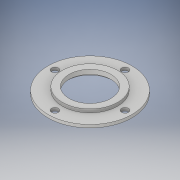
# Autodesk Inventor part: Flange_1
Saved by Autodesk Inventor 2019.4 (Build 234330000, 330)
## iProperties
Created: 2021-01-08
Part Number: Flange_1
Material: Generic
Document SubType Name: Modeling
Designer: caleb
Density: 1 g/cm^3
Appearance: Default
Author: caleb
Autodesk Inventor part; units mm, degrees
ref_plane "YZ Plane" through (0, 0, 0) normal (1, 0, 0) x (0, 1, 0)
ref_plane "XZ Plane" through (0, 0, 0) normal (0, 1, 0) x (-1, 0, 0)
ref_plane "XY Plane" through (0, 0, 0) normal (0, 0, 1) x (1, 0, 0)
sketch "Sketch1" plane through (0, 0, 0) normal (0, 1, 0) x (-1, 0, 0)
  circle A0 centre (0, 0) radius 14.2748
  dimension "d0" = 28.5496
  constraints: 1 centre point, 1 coincident
  measures "d0" diameter of A0
extrude "Extrusion1" add sketch "Sketch1" along normal blind 2.1336
sketch "Sketch2" plane through (0, 2.1336, 0) normal (0, 1, 0) x (1, 0, 0)
  circle A0 centre (0, 0) radius 9.4107
  circle A1 centre (0, 0) radius 14.2748 projected
  dimension "d3" = 18.8214
  constraints: 1 centre point, 1 coincident
  measures "d3" diameter of A0
extrude "Extrusion2" cut sketch "Sketch2" against normal blind 1.1176
sketch "Sketch3" plane through (0, 2.1336, 0) normal (0, 1, 0) x (1, 0, 0)
  circle A0 centre (0, 0) radius 7.112
  dimension "d6" = 14.224
  constraints: 1 centre point, 1 coincident
  measures "d6" diameter of A0
extrude "Extrusion3" cut sketch "Sketch3" against normal through all
chamfer "Chamfer1" distance 0.635 angle 45 1 edges at (-7.112, 0, 0)
sketch "Sketch4" plane through (0, 1.016, 0) normal (0, 1, 0) x (1, 0, 0)
  circle A0 centre (0, 0) radius 11.8999
  circle A1 centre (-11.8999, 0) radius 1.1811
  circle A2 centre (0, -11.8999) radius 1.1811
  circle A3 centre (11.8999, 0) radius 1.1811
  circle A4 centre (0, 11.8999) radius 1.1811
  dimension "d12" = 23.7998
  dimension "d13" = 2.3622
  dimension "d16" = 360
  constraints: 4 centre point, 1 coincident, 1 horizontal alignment, 11 other
  measures "d13" diameter of A1
extrude "Extrusion4" cut sketch "Sketch4" against normal through all contours A0 A3 | A0 A3 | A4 A0 | A0 A4 | A2 A0 | A0 A2 | A1 A0 | A0 A1
body "Solid1"
